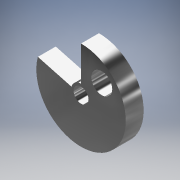
# Autodesk Inventor part: cam
Saved by Autodesk Inventor 2018.1 (Build 221171000, 171)
## iProperties
Created: 2013-08-27
Part Number: cam
Material: Generic
Document SubType Name: Modeling
Designer: Konstantin
Density: 1 g/cm^3
Appearance: Default
Mass: 0.667651 g
Surface Area: 6.8851 cm^2
Volume: 0.667651 cm^3
Author: Konstantin
Autodesk Inventor part; units mm, degrees
ref_plane "YZ Plane" through (0, 0, 0) normal (1, 0, 0) x (0, 1, 0)
ref_plane "XZ Plane" through (0, 0, 0) normal (0, 1, 0) x (-1, 0, 0)
ref_plane "XY Plane" through (0, 0, 0) normal (0, 0, 1) x (1, 0, 0)
sketch "Sketch1" plane through (0, 0, 0) normal (0, 0, 1) x (1, 0, 0)
  circle A0 centre (0, 0) radius 1.5
  arc A1 (-8.6933, 2.3294) -> (0, 9) centre (0, 0) ccw
  line L0 (0, 2) -> (0, 9)
  line L1 (-1.9319, 0.5176) -> (-8.6933, 2.3294)
  arc A2 (0, 2) -> (-1.9319, 0.5176) centre (0, 0) ccw
  constraints: 4 end point, 4 point on circle, 3 centre point, 2 vertical, 4 other
extrude "Extrusion1" add sketch "Sketch1" along normal blind 3.6
sketch "Sketch2" plane through (0, 0, 3.6) normal (0, 0, 1) x (1, 0, 0)
  circle A0 centre (4.1719, 4.1719) radius 2.1
  constraints: 1 centre point, 1 other
extrude "Extrusion2" cut sketch "Sketch2" against normal blind 3
body "Solid1"
